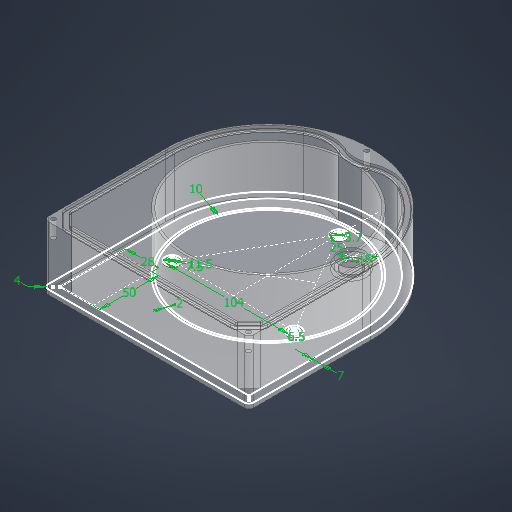
# Autodesk Inventor part: camera_base
Saved by Autodesk Inventor 2026.2 (Build 302298000, 298)
## iProperties
Created: 2026-02-25
Part Number: camera_base
Material: PET Plastic
Document SubType Name: Modeling
Designer: Tathagata Sikdar
Density: 1.541 g/cm^3
Appearance: Polycarbonate - Clear
Author: Tathagata Sikdar
Autodesk Inventor part; units mm, degrees
ref_plane "YZ Plane" through (0, 0, 0) normal (1, 0, 0) x (0, 1, 0)
ref_plane "XZ Plane" through (0, 0, 0) normal (0, 1, 0) x (-1, 0, 0)
ref_plane "XY Plane" through (0, 0, 0) normal (0, 0, 1) x (1, 0, 0)
sketch "Sketch1" plane through (0, 0, 0) normal (0, 1, 0) x (-1, 0, 0)
  line L0 (0, -60.0444) -> (52, 30.0222) construction
  line L1 (52, 30.0222) -> (-52, 30.0222) construction
  line L2 (-52, 30.0222) -> (0, -60.0444) construction
  line L3 (-26, -15.0111) -> (52, 30.0222) construction
  line L4 (0, -60.0444) -> (0, 30.0222) construction
  circle A0 centre (0, -60.0444) radius 1.85
  circle A1 centre (-52, 30.0222) radius 1.85
  circle A2 centre (52, 30.0222) radius 1.85
  circle A3 centre (0, 0) radius 68.3944
  line L5 (87.3944, 0) -> (87.3944, 100.0128)
  line L6 (-87.3944, 0) -> (-87.3944, 100.0128)
  line L7 (83.3944, 104.0128) -> (-83.3944, 104.0128)
  circle A4 centre (52, 30.0222) radius 5.75
  circle A5 centre (52, 30.0222) radius 3.75
  circle A6 centre (-52, 30.0222) radius 3.75
  circle A7 centre (-52, 30.0222) radius 5.75
  circle A8 centre (0, -60.0444) radius 3.75
  circle A9 centre (0, -60.0444) radius 5.75
  arc A10 (-87.3944, 0) -> (87.3944, 0) centre (0, 0) ccw
  arc A11 (87.3944, 100.0128) -> (83.3944, 104.0128) centre (83.3944, 100.0128) ccw
  arc A12 (-83.3944, 104.0128) -> (-87.3944, 100.0128) centre (-83.3944, 100.0128) ccw
  circle A13 centre (0, 0) radius 70.3944
  line L8 (80.3944, 97.0128) -> (52.3944, 97.0128) construction
  line L9 (52.3944, 97.0128) -> (52.3944, 47.0128) construction
  line L10 (52.3944, 47.0128) -> (80.3944, 47.0128) construction
  line L11 (80.3944, 47.0128) -> (80.3944, 97.0128) construction
  line L12 (-80.3944, 97.0128) -> (80.3944, 97.0128)
  line L13 (80.3944, 97.0128) -> (80.3944, 0)
  arc A14 (-80.3944, 0) -> (80.3944, 0) centre (0, 0) ccw
  line L14 (-80.3944, 0) -> (-80.3944, 97.0128)
  line L15 (0, -60.0444) -> (-22.2051, -48.5582) construction
  line L16 (-22.2051, -48.5582) -> (-28.4431, -62.1996) construction
  point P0 (0, -87.3944)
  point P1 (0, -68.3944)
  dimension "d0" = 3.7
  dimension "d1" = 104
  dimension "d2" = 6.5
  dimension "d28" = 11.5
  dimension "d29" = 7.5
  dimension "d70" = 4
  dimension "d172" = 50
  dimension "d173" = 28
  dimension "d205" = 2
  dimension "d206" = 7
  dimension "d207" = 10
  dimension "d262" = 25
  dimension "d263" = 15
  constraints: 34 end point, 14 centre point, 12 coincident, 11 point on circle, 7 equal radius, 6 point on line, 6 tangent, 3 horizontal, 2 collinear, 2 equal length, 2 midpoint, 2 parallel, 2 vertical, 1 line through centre, 1 perpendicular, 1 vertical alignment, 8 other
  measures "d0" diameter of A0
  measures "d1" distance of L0.end L1.end
  measures "d28" diameter of A4
  measures "d29" diameter of A5
  measures "d70" radius of A11
  measures "d172" distance of L8.end L9.end
  measures "d173" distance of L9.end L10.end
  measures "d206" distance between parallel lines of L6 L14
  measures "d262" distance of L15.start L15.end
  measures "d263" distance of L15.end L16.end
extrude "Extrusion3" add sketch "Sketch1" against normal blind 4 contours A3 | A10 L6 A12 L7 A11 L5 | A4 | A5 | A6 | A7 | A8 | A9 | A13 | L12 L13 A14 L14
extrude "Extrusion4" cut sketch "Sketch1" against normal blind 1.19 contours A4 | A7 | A9
fillet "Fillet1" radius 0.15 6 edges at (5.75, 0, -60.0444) (-46.25, 0, 30.0222) (57.75, 0, 30.0222) (3.75, 0, -60.0444) (55.75, 0, 30.0222) (-48.25, 0, 30.0222)
fillet "Fillet2" radius 0.25 3 edges at (5.75, -1.19, -60.0444) (57.75, -1.19, 30.0222) (-46.25, -1.19, 30.0222)
extrude "Extrusion6" add sketch "Sketch1" along normal blind 50 contours A13
extrude "Extrusion19" add sketch "Sketch1" along normal up to surface (50 mm away) contours A10 L6 A12 L7 A11 L5
sketch "Sketch16" plane through (0, 50, 0) normal (0, 1, 0) x (1, 0, 0)
  circle A0 centre (-83.3944, -100.0128) radius 1.85
  arc A1 (87.3944, 0) -> (-87.3944, 0) centre (0, 0) ccw construction
  line L0 (-87.3944, -100.0128) -> (-87.3944, 0) construction
  arc A2 (-87.3944, -100.0128) -> (-83.3944, -104.0128) centre (-83.3944, -100.0128) ccw construction
  line L1 (83.3944, -104.0128) -> (-83.3944, -104.0128) construction
  arc A3 (83.3944, -104.0128) -> (87.3944, -100.0128) centre (83.3944, -100.0128) ccw construction
  line L2 (87.3944, 0) -> (87.3944, -100.0128) construction
  circle A4 centre (83.3944, -100.0128) radius 1.85
  circle A5 centre (0, 83.8944) radius 1.85
  arc A6 (80.3944, 0) -> (-80.3944, 0) centre (0, 0) ccw construction
  line L3 (-80.3944, 0) -> (-80.3944, -97.0128) construction
  arc A7 (-10, 69.6805) -> (-39.9607, 69.7596) centre (-25.049, 43.7281) ccw
  arc A8 (39.9607, 69.7596) -> (10, 69.6805) centre (25.049, 43.7281) ccw
  arc A9 (39.9607, 69.7596) -> (-39.9607, 69.7596) centre (0, 0) ccw
  line L4 (0, 80.3944) -> (0, 83.8944) construction
  arc A10 (10, 69.6805) -> (-10, 69.6805) centre (0, 0) ccw
  circle A11 centre (0, 0) radius 70.3944 construction
  point P0 (-80.3944, -90.6836)
  dimension "M4Hole" = 3.7
  dimension "d215" = 3.5
  dimension "d241" = 30
  dimension "d242" = 20
  constraints: 15 point on circle, 7 centre point, 5 equal radius, 2 coincident, 2 end point, 2 tangent, 1 symmetric about line, 1 vertical, 1 vertical alignment
  measures "M4Hole" diameter of A4
  measures "d215" distance of point (0, 80.394) L4.end
  measures "d241" radius of A8
  measures "d242" distance of A8.end A7.start
extrude "Extrusion22" add sketch "Sketch16" against normal up to surface (50 mm away) contours A7 A9 A8 A10
chamfer "Chamfer6" distance 10 angle 45 1 edges at (-80.3944, 25, 97.0128) measured on face at (-80.3944, 25, 96.5128)
chamfer "Chamfer7" distance 10 angle 45 1 edges at (80.3944, 25, 97.0128) measured on face at (79.8944, 25, 97.0128)
extrude "Extrusion23" cut sketch "Sketch16" against normal blind 14 contours A0 | A4 | A5
sketch "Sketch17" plane through (0, 50, 0) normal (0, 1, 0) x (1, 0, 0)
  circle A0 centre (-83.3944, -100.0128) radius 1.85 construction
  circle A1 centre (83.3944, -100.0128) radius 1.85 construction
  circle A2 centre (0, 83.8944) radius 1.85 construction
  arc A3 (87.3944, 0) -> (-87.3944, 0) centre (0, 0) ccw construction
  line L0 (-87.3944, -100.0128) -> (-87.3944, 0) construction
  arc A4 (-87.3944, -100.0128) -> (-83.3944, -104.0128) centre (-83.3944, -100.0128) ccw construction
  line L1 (83.3944, -104.0128) -> (-83.3944, -104.0128) construction
  arc A5 (83.3944, -104.0128) -> (87.3944, -100.0128) centre (83.3944, -100.0128) ccw construction
  line L2 (87.3944, 0) -> (87.3944, -100.0128) construction
  arc A6 (-10, 69.6805) -> (10, 69.6805) centre (0, 0) ccw construction
  arc A7 (39.9607, 69.7596) -> (10, 69.6805) centre (25.049, 43.7281) ccw construction
  arc A8 (80.3944, 0) -> (39.9607, 69.7596) centre (0, 0) ccw construction
  line L3 (80.3944, -87.0128) -> (80.3944, 0) construction
  line L4 (70.3944, -97.0128) -> (80.3944, -87.0128) construction
  line L5 (-70.3944, -97.0128) -> (70.3944, -97.0128) construction
  line L6 (-80.3944, -87.0128) -> (-70.3944, -97.0128) construction
  line L7 (-80.3944, 0) -> (-80.3944, -87.0128) construction
  arc A9 (-39.9607, 69.7596) -> (-80.3944, 0) centre (0, 0) ccw construction
  arc A10 (-10, 69.6805) -> (-39.9607, 69.7596) centre (-25.049, 43.7281) ccw construction
  circle A11 centre (0, 0) radius 68.3944 construction
  arc A12 (-12.2349, 72.4164) -> (-40.6666, 70.9918) centre (-25.049, 43.7281) ccw
  arc A13 (-40.6666, 70.9918) -> (-81.8144, 0) centre (0, 0) ccw
  line L8 (-81.8144, 0) -> (-81.8144, -86.7725)
  line L9 (-81.2286, -88.1867) -> (-71.5684, -97.847)
  line L10 (-70.1542, -98.4328) -> (70.1542, -98.4328)
  line L11 (71.5684, -97.847) -> (81.2286, -88.1867)
  line L12 (81.8144, -86.7725) -> (81.8144, 0)
  arc A14 (81.8144, 0) -> (40.6666, 70.9918) centre (0, 0) ccw
  arc A15 (40.6666, 70.9918) -> (12.2349, 72.4164) centre (25.049, 43.7281) ccw
  arc A16 (-12.2349, 72.4164) -> (12.2349, 72.4164) centre (0, 99.8081) ccw
  arc A17 (-81.8144, -86.7725) -> (-81.2286, -88.1867) centre (-79.8144, -86.7725) ccw
  arc A18 (-71.5684, -97.847) -> (-70.1542, -98.4328) centre (-70.1542, -96.4328) ccw
  arc A19 (70.1542, -98.4328) -> (71.5684, -97.847) centre (70.1542, -96.4328) ccw
  arc A20 (81.2286, -88.1867) -> (81.8144, -86.7725) centre (79.8144, -86.7725) ccw
  arc A21 (85.9744, 0) -> (42.7343, 74.6015) centre (0, 0) ccw
  line L13 (85.9744, 0) -> (85.9744, -86.7725)
  arc A22 (84.1702, -91.1283) -> (85.9744, -86.7725) centre (79.8144, -86.7725) ccw
  line L14 (84.1702, -91.1283) -> (74.51, -100.7885)
  arc A23 (70.1542, -102.5928) -> (74.51, -100.7885) centre (70.1542, -96.4328) ccw
  line L15 (70.1542, -102.5928) -> (-70.1542, -102.5928)
  arc A24 (-74.51, -100.7885) -> (-70.1542, -102.5928) centre (-70.1542, -96.4328) ccw
  line L16 (-74.51, -100.7885) -> (-84.1702, -91.1283)
  arc A25 (-85.9744, -86.7725) -> (-84.1702, -91.1283) centre (-79.8144, -86.7725) ccw
  line L17 (-85.9744, -86.7725) -> (-85.9744, 0)
  arc A26 (-42.7343, 74.6015) -> (-85.9744, 0) centre (0, 0) ccw
  arc A27 (-10.5384, 76.2147) -> (-42.7343, 74.6015) centre (-25.049, 43.7281) ccw
  arc A28 (-10.5384, 76.2147) -> (10.5384, 76.2147) centre (0, 99.8081) ccw
  arc A29 (42.7343, 74.6015) -> (10.5384, 76.2147) centre (25.049, 43.7281) ccw
  dimension "d253" = 2
  dimension "d254" = 30
  dimension "GasketWidth" = 4.16
  dimension "d256" = 7
  dimension "d257" = 1.42
  constraints: 36 point on circle, 20 end point, 18 centre point, 10 tangent, 3 equal radius, 21 other
  measures "d253" radius of A17
  measures "d254" radius of A16
  measures "GasketWidth" distance between parallel lines of L12 L13
  measures "d256" distance between parallel lines of L2 L3
  measures "d257" distance between parallel lines of L12 L3
extrude "Extrusion24" cut sketch "Sketch17" against normal blind 2.38
fillet "Fillet7" radius 0.2 28 edges at (26.8295, 47.62, -79.2635) (74.383, 47.62, -43.1135) (85.9744, 47.62, 43.3863) (85.5055, 47.62, 89.1298) (79.3401, 47.62, 95.9584) (72.5115, 47.62, 102.1239) (0, 47.62, 102.5928) (-72.5115, 47.62, 102.1239) (-79.3401, 47.62, 95.9584) (-85.5055, 47.62, 89.1298) (-85.9744, 47.62, 43.3863) (-74.383, 47.62, -43.1135) (-26.8295, 47.62, -79.2635) (0, 47.62, -73.9681) (-26.6213, 47.62, -75.1087) (-70.7839, 47.62, -41.0274) (-81.8144, 47.62, 43.3863) (-81.6622, 47.62, 87.5379) (-76.3985, 47.62, 93.0168) (-70.9196, 47.62, 98.2805) (0, 47.62, 98.4328) (70.9196, 47.62, 98.2805) (76.3985, 47.62, 93.0168) (81.6622, 47.62, 87.5379) (81.8144, 47.62, 43.3863) (70.7839, 47.62, -41.0274) (26.6213, 47.62, -75.1087) (0, 47.62, -69.8081)
hole "Hole2" at (22.2051, 0, -48.5582) direction (0, -1, 0) diameter 21 end through all
sketch "Sketch18" plane through (0, -4, 0) normal (0, -1, 0) x (1, 0, 0)
  circle A0 centre (22.2051, -48.5582) radius 10.5 projected
  circle A1 centre (22.2051, -48.5582) radius 12.5
  point P0 (0, 0)
  dimension "d271" = 2
  constraints: 1 centre point, 1 coincident
  measures "d271" radial gap between concentric circles of A1 A0
extrude "Extrusion25" add sketch "Sketch18" along normal blind 4.5
sketch "Sketch19" plane through (22.2051, -8.5, -48.5582) normal (0, -1, 0) x (1, 0, 0)
  circle A0 centre (0, 0) radius 12.5 projected
  circle A1 centre (0, 0) radius 8
  point P0 (-22.2051, 48.5582)
  dimension "d274" = 16
  constraints: 1 centre point, 1 coincident
  measures "d274" diameter of A1
extrude "Extrusion26" add sketch "Sketch19" against normal blind 1
body "Solid3"
